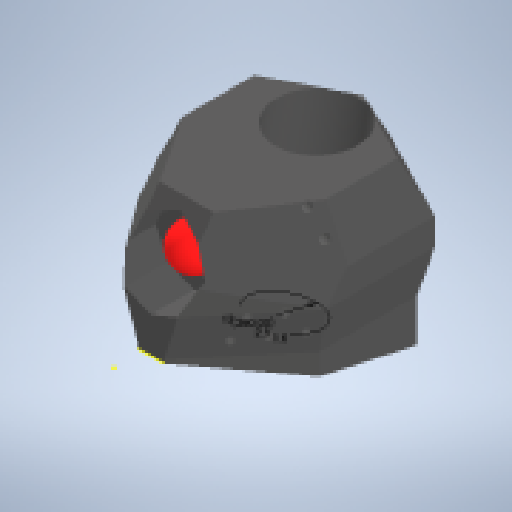
# Autodesk Inventor part: head_bace
Saved by Autodesk Inventor 2026.1 (Build 301233020, 233B)
## iProperties
Created: 2024-02-25
Part Number: head_bace
Material: 一般
Document SubType Name: Modeling
Designer: hibik
Density: 1 g/cm^3
Appearance: 既定
Author: hibik
Autodesk Inventor part; units mm, degrees
sketch "スケッチ1" plane through (0, 0, 0) normal (0, 1, 0) x (-1, 0, 0)
  line L0 (-17.5, -21) -> (0, 0)
  line L1 (0, 0) -> (17.5, -21)
  line L2 (17.5, -21) -> (17.5, -41)
  line L3 (17.5, -41) -> (0, -50)
  line L4 (0, -50) -> (-17.5, -41)
  line L5 (-17.5, -41) -> (-17.5, -21)
  line L6 (0, -60) -> (0, 10) projected
  line L7 (24.5, 0) -> (-24.5, 0) projected
  dimension "d0" = 50
  dimension "d12" = 35
  dimension "d13" = 20
  dimension "d14" = 21
  constraints: 12 end point, 2 horizontal alignment, 1 coincident, 1 point on line, 1 vertical, 2 other
  measures "d0" distance of L0.end L3.end
  measures "d12" distance between parallel lines of L5 L2
  measures "d13" distance of L4.end L0.start
  measures "d14" vertical distance of L0.end L1.end
extrude "押し出し1" add sketch "スケッチ1" along normal blind 18
chamfer "面取り1" distance 5 distance2 10 6 edges at (8.75, 18, -10.5) (17.5, 18, -31) (8.75, 18, -45.5) (-8.75, 18, -45.5) (-17.5, 18, -31) (-8.75, 18, -10.5) measured on face at (0, 18, -30.6667)
extrude "押し出し2" add sketch "スケッチ1" against normal blind 5
ref_plane "作業平面1" through (0, 8, 0) normal (0, -0.7881104, 0.6155339) x (1, 0, 0)
sketch "スケッチ2" plane through (0, 8, 0) normal (0, -0.7881104, 0.6155339) x (1, 0, 0)
  line L0 (0, 0) -> (17.5, -16.550319)
  line L1 (-17.5, -16.550319) -> (0, 0)
  line L2 (-5, -4.728662) -> (-5, -4.728662)
  line L3 (-5, -4.728662) -> (5, -4.728662)
  line L4 (13.334597, -12.610962) -> (5, -4.728662)
  line L5 (-5, -4.728662) -> (-23.641343, -26.94455)
  line L6 (5, -4.728662) -> (18.717304, -21.076309)
  line L7 (-23.641343, -26.94455) -> (-26.210864, -24.788466)
  line L8 (-26.210864, -24.788466) -> (-17.5, -16.550319)
  line L9 (17.5, -16.550319) -> (23.817771, -21.851558)
  line L10 (23.817771, -21.851558) -> (18.717304, -21.076309)
  point P0 (0, -4.924271)
  dimension "d9" = 10
  dimension "d25" = 130
  dimension "d26" = 130
  constraints: 18 end point, 4 point on line, 2 collinear, 1 horizontal, 1 parallel
  measures "d9" distance of L2.end L3.end
  measures "d25" angle of L3 L5
  measures "d26" angle of L6 L3
extrude "押し出し3" cut sketch "スケッチ2" against normal through all
chamfer "面取り2" distance 2 distance2 8 6 edges at (-8.75, -5, -10.5) (-17.5, -5, -31) (-8.75, -5, -45.5) (8.75, -5, -45.5) (17.5, -5, -31) (8.75, -5, -10.5) measured on face at (0, -5, -30.6667)
sketch "スケッチ3" plane through (0, -5, 0) normal (0, -1, 0) x (1, 0, 0)
  line L0 (0, -3.1241) -> (15.5, -21.7241)
  line L1 (-15.5, -21.7241) -> (0, -3.1241)
  line L2 (-15.5, -39.779581) -> (-15.5, -21.7241)
  line L3 (0, -47.751009) -> (-15.5, -39.779581)
  line L4 (15.5, -39.779581) -> (0, -47.751009)
  line L5 (15.5, -21.7241) -> (15.5, -39.779581)
  point P0 (0, 0)
extrude "押し出し4" add sketch "スケッチ3" along normal blind 8
ref_plane "作業平面2" through (0, -5, -3.1241) normal (0, -0.9770022, 0.2132292) x (-0.3818297, -0.1970734, -0.9029774)
sketch "スケッチ4" plane through (0, -5, -3.1241) normal (0, -0.9770022, 0.2132292) x (-0.3818297, -0.1970734, -0.9029774)
  line L0 (80, -28.484839) -> (-10, -28.484839)
  line L1 (-10, -28.484839) -> (-10, 40)
  line L2 (-10, 40) -> (80, 40)
  line L3 (80, 40) -> (80, -28.484839)
  point P0 (-3.806358, -1.572527)
  constraints: 8 end point, 2 parallel, 1 horizontal, 1 perpendicular
extrude "押し出し5" cut sketch "スケッチ4" along normal through all
ref_plane "作業平面3" through (-5, 8, -6) normal (0, 0, 1) x (1, 0, 0)
sketch "スケッチ5" plane through (-5, 8, -6) normal (0, 0, 1) x (1, 0, 0)
  line L0 (-30, 20) -> (40, 20)
  line L1 (40, 20) -> (40, -30)
  line L2 (40, -30) -> (-30, -30)
  line L3 (-30, -30) -> (-30, 20)
  point P0 (5, -8)
  constraints: 8 end point, 2 parallel, 1 horizontal, 1 perpendicular
extrude "押し出し6" cut sketch "スケッチ5" along normal through all
sketch "スケッチ6" plane through (-5, 8, -6) normal (0, 0, 1) x (1, 0, 0)
  line L0 (0, 0) -> (10, 0)
  circle A0 centre (5, 0) radius 5
  line L1 (9.949747, -4.949747) -> (5, -7)
  line L2 (5, -7) -> (0.050253, -4.949747)
  line L3 (0.050253, -4.949747) -> (-2, 0)
  line L4 (-2, 0) -> (0.050253, 4.949747)
  line L5 (0.050253, 4.949747) -> (5, 7)
  line L6 (5, 7) -> (9.949747, 4.949747)
  line L7 (9.949747, 4.949747) -> (12, 0)
  line L8 (12, 0) -> (9.949747, -4.949747)
  point P0 (5, -8)
  dimension "d29" = 7
  constraints: 16 end point, 2 midpoint, 1 coincident, 1 horizontal alignment, 1 vertical alignment, 19 other
  measures "d29" distance of point (5, 0) L5.end
extrude "押し出し7" cut sketch "スケッチ6" against normal blind 8 contours A0 L0 | L0 A0 | L1 L2 L3 L4 L5 L6 L7 L8
sketch "スケッチ8" plane through (-5, 8, -14) normal (0, 0, 1) x (1, 0, 0)
  line L0 (5, 0) -> (-12.5, 0) projected
  circle A0 centre (5, 0) radius 4
  line L1 (5, 4) -> (5, -4)
  line L2 (5, -5) -> (5, 0) projected
  point P0 (5, -8)
  dimension "d32" = 8
  constraints: 2 end point, 2 point on circle, 1 centre point, 1 midpoint, 1 point on line
  measures "d32" diameter of A0
revolve "回転1" add sketch "スケッチ8" angle 360 about axis through (0, 12, -14) along (0, -1, 0) contours L1 A0
sketch "スケッチ9" plane through (-15.5, -5, -21.7241) normal (-0.7452841, -0.2425356, 0.6210701) x (0.6214323, 0.0848617, 0.7788584)
  circle A0 centre (10.296176, 6.656412) radius 0.8
  circle A1 centre (12.004779, 1.957404) radius 0.8
  circle A2 centre (7.081017, 2.827215) radius 0.8
  circle A3 centre (2.157255, 3.697026) radius 0.8
  circle A4 centre (5.372415, 7.526223) radius 0.8
  line L0 (2.157255, 3.697026) -> (7.081017, 2.827215) construction
  line L1 (7.081017, 2.827215) -> (12.004779, 1.957404) construction
  line L2 (12.004779, 1.957404) -> (7.081017, 2.827215)
  line L3 (5.372415, 7.526223) -> (10.296176, 6.656412) construction
  line L4 (10.296176, 6.656412) -> (9.542898, 2.39231) construction
  line L5 (5.372415, 7.526223) -> (4.619136, 3.262121) construction
  line L6 (10.296176, 6.656412) -> (12.004779, 1.957404) construction
  line L7 (12.004779, 1.957404) -> (11.737934, 0.44687) construction
  line L8 (12.004779, 1.957404) -> (13.292724, 2.425713) construction
  line L9 (20.389733, -1.790423) -> (19.45078, 6.569969)
  line L10 (0, 0) -> (20.389733, -1.790423)
  point P0 (26.976506, 2.987508)
  dimension "d34" = 1.6
  dimension "d35" = 5
  dimension "d36" = 5
  dimension "d37" = 7.91428
  dimension "d38" = 3
  constraints: 18 end point, 5 centre point, 4 equal radius, 4 perpendicular, 3 equal length, 2 midpoint, 1 collinear
  measures "d34" diameter of A1
  measures "d35" distance from line of L0.end L7
  measures "d36" distance from line of L3.end L8
  measures "d37" distance from line of L9 L1.end
  measures "d38" distance from line of L10 L1.end
extrude "押し出し8" cut sketch "スケッチ9" against normal blind 5
sketch "スケッチ10" plane through (-12.5, 18, -25.151493) normal (-0.7660444, 0.3956576, 0.5065876) x (0.5515991, 0, 0.8341093)
  circle A0 centre (2.173773, -2.388026) radius 0.8
  circle A1 centre (0.208151, -6.893534) radius 0.8
  point P0 (27.874085, -17.895067)
extrude "押し出し9" cut sketch "スケッチ10" against normal blind 5
mirror "ミラー1" about plane through (0, 0, 0) normal (1, 0, 0) of "押し出し8", "押し出し9"
sketch "スケッチ11" plane through (0, -5, -3.1241) normal (0, -0.9770022, 0.2132292) x (0.9242327, -0.0814172, -0.3730484)
  line L0 (3.338953, -1.805481) -> (-1.091048, -3.635655)
  line L1 (-7.0564, -23.513743) -> (-1.091048, -3.635655)
  line L2 (0, -40.594018) -> (-7.0564, -23.513743)
  line L3 (28.651214, -28.757298) -> (0, -40.594018)
  line L4 (21.594814, -11.677024) -> (28.651214, -28.757298)
  line L5 (3.338953, -1.805481) -> (21.594814, -11.677024)
  line L6 (0, -40.594018) -> (21.594814, -11.677024)
  line L7 (-7.0564, -23.513743) -> (28.651214, -28.757298)
  circle A0 centre (10.797407, -26.135521) radius 4.25
  point P0 (-1.572527, 3.806358)
  dimension "d43" = 8.5
  constraints: 4 end point, 1 centre point, 1 midpoint
  measures "d43" diameter of A0
ref_plane "作業平面4" through (0, -10.052708, -30.965069) normal (0, -0.9770022, 0.2132292) x (1, 0, 0)
sketch "スケッチ12" plane through (0, -10.052708, -30.965069) normal (0, -0.9770022, 0.2132292) x (1, 0, 0)
  circle A0 centre (0, 0) radius 4.25 projected
  circle A1 centre (0, 0) radius 0.8
  point P0 (0, 32.396472)
  dimension "d46" = 1.6
  constraints: 1 centre point, 1 coincident
  measures "d46" diameter of A1
extrude "押し出し11" cut sketch "スケッチ12" against normal blind 5 contours A1
sketch "スケッチ13" plane through (0, 18, 0) normal (0, 1, 0) x (1, 0, 0)
  line L0 (-30, 50) -> (40, 50)
  line L1 (40, 50) -> (40, 0)
  line L2 (40, 0) -> (-30, 0)
  line L3 (-30, 0) -> (-30, 50)
  point P0 (0, 0)
  constraints: 8 end point, 2 parallel, 1 horizontal, 1 perpendicular
extrude "押し出し12" cut sketch "スケッチ13" against normal blind 1.5
sketch "スケッチ14" plane through (0, -5, -3.1241) normal (0, -0.9770022, 0.2132292) x (0.9242327, -0.0814172, -0.3730484)
  circle A0 centre (10.797407, -26.135521) radius 0.8
  circle A1 centre (10.797407, -26.135521) radius 6 construction
  circle A2 centre (8.506429, -20.590124) radius 0.8
  line L0 (3.338953, -1.805481) -> (-1.091048, -3.635655)
  line L1 (1.123952, -2.720568) -> (10.797407, -26.135521) construction
  circle A3 centre (5.256254, -23.834299) radius 0.8
  circle A4 centre (5.252011, -28.426499) radius 0.8
  circle A5 centre (8.496186, -31.676674) radius 0.8
  circle A6 centre (13.088385, -31.680917) radius 0.8
  circle A7 centre (16.338561, -28.436742) radius 0.8
  circle A8 centre (16.342804, -23.844543) radius 0.8
  circle A9 centre (13.098628, -20.594367) radius 0.8
  circle A10 centre (10.797407, -26.135521) radius 8.5
  point P0 (-1.572527, 3.806358)
  dimension "d51" = 12
  dimension "d52" = 1.6
  dimension "d55" = 360
  dimension "d57" = 2.5
  constraints: 9 centre point, 2 coincident, 2 end point, 1 midpoint, 1 perpendicular, 1 point on line, 20 other
  measures "d52" diameter of A2
sketch "スケッチ14 outline for 押し出し13" plane through (0, -5, -3.1241) normal (0, -0.9770022, 0.2132292) x (0.9242327, -0.0814172, -0.3730484)
  circle A0 centre (10.797407, -26.135521) radius 8.5
extrude "押し出し13" cut sketch "スケッチ14 outline for 押し出し13" against normal up to surface draft -2 surface through (5, 16.5, -25) normal (0, -1, 0)
extrude "押し出し14" add sketch "スケッチ14" against normal blind 5
